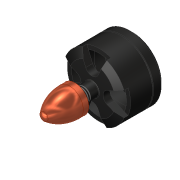
# Autodesk Inventor part: EMAX_MT1806
Saved by Autodesk Inventor 2019 (Build 230136000, 136)
## iProperties
Created: 2022-04-03
Part Number: EMAX_MT1806
Material: Steel, Alloy
Document SubType Name: Modeling
Designer: solyo
Density: 7.73 g/cm^3
Appearance: Glossy - Black
Mass: 24.6545 g
Surface Area: 38.023 cm^2
Volume: 3.18946 cm^3
Author: solyo
Autodesk Inventor part; units mm, degrees
ref_plane "YZ Plane" through (0, 0, 0) normal (1, 0, 0) x (0, 1, 0)
ref_plane "XZ Plane" through (0, 0, 0) normal (0, 1, 0) x (-1, 0, 0)
ref_plane "XY Plane" through (0, 0, 0) normal (0, 0, 1) x (1, 0, 0)
sketch "Sketch1" plane through (0, 0, 0) normal (0, 0, 1) x (1, 0, 0)
  circle A0 centre (0, 0) radius 11.5
  dimension "d0" = 23
  constraints: 1 centre point, 1 coincident
  measures "d0" diameter of A0
extrude "Extrusion1" add sketch "Sketch1" along normal blind 14.7
sketch "Sketch2" plane through (0, 0, 14.7) normal (0, 0, 1) x (1, 0, 0)
  circle A0 centre (0, 0) radius 2.5
  dimension "d3" = 5
  constraints: 1 centre point, 1 coincident
  measures "d3" diameter of A0
extrude "Extrusion2" add sketch "Sketch2" along normal blind 10
thread "Thread1" size "M5x0.8" class "6g" standard "ANSI Metric M Profile" length 7
sketch "Sketch3" plane through (0, 0, 0) normal (0, 0, -1) x (-1, 0, 0)
  circle A0 centre (0, 0) radius 1
  dimension "d8" = 2
  constraints: 1 centre point, 1 coincident
  measures "d8" diameter of A0
extrude "Extrusion3" add sketch "Sketch3" along normal blind 2 separate body
ref_plane "Work Plane1" through (0, 0, 4) normal (0, 0, -1) x (-1, 0, 0)
split body "Split1" result two bodies by plane through (0, 0, 4) normal (0, 0, -1) bodies 1 first body at (-0.5734, -2.888, 3.5)
chamfer "Chamfer1" distance 3 distance2 1 1 edges at (-11.5, 0, 14.7) measured on face at (-11, 0, 14.7)
chamfer "Chamfer2" distance 1 angle 45 1 edges at (-11.5, 0, 0)
sketch "Sketch4" plane through (0, 0, 14.7) normal (0, 0, 1) x (1, 0, 0)
  line L0 (-4.3682, 10.6381) -> (-2.318, 5.5635)
  arc A0 (-2.318, 5.5635) -> (2.318, 5.5635) centre (0, 6.5) ccw
  line L1 (2.318, 5.5635) -> (4.3682, 10.6381)
  line L2 (0, 0) -> (0, 4.4221) construction
  circle A1 centre (0, 0) radius 2.5 projected
  circle A2 centre (0, 0) radius 11.5 projected
  circle A3 centre (0, 0) radius 8.5 projected
  dimension "d12" = 22
  dimension "d13" = 22
  dimension "d14" = 2.5
  dimension "d15" = 6.5
  constraints: 6 end point, 4 point on circle, 2 tangent, 1 centre point, 1 vertical, 1 vertical alignment
  measures "d12" angle of L2 L0
  measures "d13" angle of L2 L1
  measures "d14" radius of A0
  measures "d15" distance of A0.centre L2.start
extrude "Extrusion4" cut sketch "Sketch4" against normal blind 2.5 contours A2 L1 A3 L0 | A3 L1 A0 L0 picked at (-0.7421, 10.4275) picked at (-1.3239, 7.467) bodies 4
pattern_circular "Circular Pattern1" count 4 over 360 about axis through (0, 0, 0) along (0, 0, 1) of "Extrusion4" bodies 4
fillet "Fillet1" radius 0.2 1 edges at (-2.5, 0, 14.7)
sketch "Sketch5" plane through (0, 0, 0) normal (0, 0, -1) x (-1, 0, 0)
  point P0 (0, 0)
  point P1 (8, 0)
  point P2 (-8, 0)
  point P3 (0, -6)
  point P4 (0, 6)
  dimension "d31" = 12
  dimension "d32" = 16
  dimension "d33" = 8
  dimension "d34" = 6
  constraints: 2 horizontal alignment, 2 vertical alignment
  measures "d31" distance of point (0, -6) point (0, 6)
  measures "d32" distance of point (-8, 0) point (8, 0)
  measures "d33" distance of point (0, 0) point (8, 0)
  measures "d34" distance of point (0, 0) point (0, 6)
hole "Hole1" at (-8, 0, 0) at (8, 0, 0) at (0, -6, 0) at (0, 6, 0) direction (0, 0, 1) diameter 1.567 depth 4 tip angle 118 bodies 3 thread size "M2x0.4" class "6H" standard "ISO Metric profile"
chamfer "Chamfer4" distance 0.2 angle 45 7 edges at (1, 0, -2) (-8, -0.7835, 0) (0, 5.2165, 0) (8, -0.7835, 0) (0, -6.7835, 0) (-11.5, 0, 4) (-2.5, 0, 24.7)
sketch "Sketch6" plane through (0, 0, 14.7) normal (0, 0, 1) x (1, 0, 0)
  circle A0 centre (0, 0) radius 1 projected
  circle A1 centre (0, 0) radius 63.5
  dimension "d45" = 127
  constraints: 1 centre point, 1 coincident
  measures "d45" diameter of A1
sketch "Sketch7" plane through (0, 0, 12.2) normal (0, 0, 1) x (1, 0, 0)
  circle A0 centre (0, 0) radius 1 projected
  circle A1 centre (0, 0) radius 10
  dimension "d46" = 20
  constraints: 1 centre point, 1 coincident
  measures "d46" diameter of A1
extrude "Extrusion5" cut sketch "Sketch7" against normal blind 12 bodies 4 3
sketch "Sketch8" plane through (0, 0, 0) normal (1, 0, 0) x (0, 1, 0)
  line L0 (-2.3, 24.7) -> (2.3, 24.7) projected
  line L1 (-2.5, 14.9) -> (2.5, 14.9) projected
  line L2 (2.5, 24.5) -> (-2.5, 24.5) projected
  line L3 (2.5, 14.9) -> (2.5, 24.5) projected
  line L4 (2.5, 20.9) -> (2.5, 25.4)
  line L5 (2.5, 25.4) -> (0, 26.8434)
  line L6 (-2.5, 14.9) -> (-2.5, 24.5) projected
  line L7 (2.5, 20.9) -> (3.1243, 20.9)
  line L8 (3.1243, 20.9) -> (5, 20.9)
  line L9 (5, 20.9) -> (5, 22.9)
  line L10 (0, 0) -> (0, 46.5668)
  arc A0 (5, 22.9) -> (1.5068, 32.2151) centre (-9.1667, 22.9) ccw
  arc A1 (1.5068, 32.2151) -> (0, 32.9) centre (0, 30.9) ccw
  line L11 (1.7734, 32.9) -> (-2.3, 32.9) construction
  dimension "d51" = 4.5
  dimension "d52" = 60
  dimension "d53" = 6
  dimension "d54" = 2
  dimension "d59" = 12
  dimension "d60" = 2
  dimension "d61" = 10
  constraints: 14 end point, 5 point on line, 4 point on circle, 3 tangent, 2 centre point, 2 horizontal, 2 vertical, 1 perpendicular, 1 vertical alignment
  measures "d51" distance of L4.start L4.end
  measures "d52" angle of L5 L10
  measures "d53" distance between parallel lines of L1 L8
  measures "d54" distance of L8.end L9.end
  measures "d59" distance between parallel lines of L11 L8
  measures "d60" radius of A1
  measures "d61" diameter of L9 L10
revolve "Revolution1" add sketch "Sketch8" angle 360 about axis through (0, 0, 0) along (0, 0, 1) separate body contours L3 L4 L5 L10 A1 A0 L9 L8 L7
equation "\"d13\" = d12"
equation "\"d33\" = 0.5 * d32"
equation "\"d34\" = 0.5 * d31"
body "Solid2"
body "Solid5"
body "Solid3"
body "Solid4"
